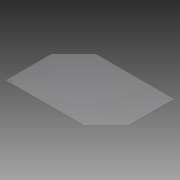
# Autodesk Inventor part: polycarb sheet
Saved by Autodesk Inventor 2015 SP1 (Build 190203100, 203)
## iProperties
Created: 2015-01-19
Part Number: polycarb sheet
Material: Polycarbonate, Clear
Document SubType Name: Modeling
Designer: Jarod
Density: 1.2 g/cm^3
Appearance: Polycarbonate - Clear
Author: Jarod
Autodesk Inventor part; units mm, degrees
ref_plane "YZ Plane" through (0, 0, 0) normal (1, 0, 0) x (0, 1, 0)
ref_plane "XZ Plane" through (0, 0, 0) normal (0, 1, 0) x (-1, 0, 0)
ref_plane "XY Plane" through (0, 0, 0) normal (0, 0, 1) x (1, 0, 0)
sketch "Sketch1" plane through (0, 0, 0) normal (0, 1, 0) x (-1, 0, 0)
  line L0 (0, 0) -> (546.1, 0)
  line L1 (546.1, 0) -> (546.1, 368.3)
  line L2 (546.1, 368.3) -> (0, 368.3)
  line L3 (0, 368.3) -> (0, 0)
  circle A0 centre (12.7, 12.7) radius 3.175
  circle A1 centre (12.7, 355.6) radius 3.175
  circle A2 centre (533.4, 355.6) radius 3.175
  circle A3 centre (533.4, 12.7) radius 3.175
  dimension "d0" = 546.1
  dimension "d1" = 368.3
  dimension "d2" = 12.7
  dimension "d3" = 12.7
  dimension "d4" = 12.7
  dimension "d5" = 12.7
  dimension "d6" = 12.7
  dimension "d7" = 12.7
  dimension "d8" = 12.7
  dimension "d9" = 12.7
  dimension "d15" = 6.35
  dimension "d16" = 6.35
  dimension "d17" = 6.35
  dimension "d19" = 6.35
  constraints: 8 end point, 4 centre point, 4 coincident, 2 parallel, 1 horizontal, 1 perpendicular
  measures "d0" distance of L2.end L1.end
  measures "d1" distance of L1.end L0.end
  measures "d2" distance from line of L0 point (12.7, 12.7)
  measures "d3" distance from line of L3 point (12.7, 12.7)
  measures "d4" distance from line of L2 point (12.7, 355.6)
  measures "d5" distance from line of L3 point (12.7, 355.6)
  measures "d6" distance from line of L2 point (533.4, 355.6)
  measures "d7" distance from line of L1 point (533.4, 355.6)
  measures "d8" distance from line of L1 point (533.4, 12.7)
  measures "d9" distance from line of L0 point (533.4, 12.7)
  measures "d15" diameter of A0
  measures "d16" diameter of A1
  measures "d17" diameter of A2
  measures "d19" diameter of A3
extrude "Extrusion3" add sketch "Sketch1" along normal blind 3.175
body "Solid2"
